Autodesk Fusion 360 part; units mm, degrees
(part 3 of 4)
sketch "Sketch5" plane through (0, 20, 0) normal (0, 1, 0) x (-1, 0, 0)
  line L0 (-11, 35) -> (-11, 37.5)
  line L1 (-11, 37.5) -> (-8.5, 37.5)
  line L2 (-8.5, 37.5) -> (-8.5, 35)
  line L3 (-8.5, 35) -> (-11, 35)
  line L4 (2.5, 35) -> (2.5, 37.5)
  line L5 (2.5, 37.5) -> (5, 37.5)
  line L6 (5, 37.5) -> (5, 35)
  line L7 (5, 35) -> (2.5, 35)
  line L8 (95, -45) -> (95, 155)
  line L9 (95, 155) -> (-95, 155)
  line L10 (-95, 155) -> (-95, -45)
  line L11 (-95, -45) -> (95, -45)
  line L12 (-63.1566, 125.0807) -> (-65.6424, 118.6138)
  line L13 (-65.6424, 118.6138) -> (-72.4858, 117.5331)
  line L14 (-72.4858, 117.5331) -> (-76.8434, 122.9193)
  line L15 (-76.8434, 122.9193) -> (-74.3576, 129.3862)
  line L16 (-74.3576, 129.3862) -> (-67.5142, 130.4669)
  line L17 (-67.5142, 130.4669) -> (-63.1566, 125.0807)
  line L18 (-63.1566, 93.0807) -> (-65.6424, 86.6138)
  line L19 (-65.6424, 86.6138) -> (-72.4858, 85.5331)
  line L20 (-72.4858, 85.5331) -> (-76.8434, 90.9193)
  line L21 (-76.8434, 90.9193) -> (-74.3576, 97.3862)
  line L22 (-74.3576, 97.3862) -> (-67.5142, 98.4669)
  line L23 (-67.5142, 98.4669) -> (-63.1566, 93.0807)
  line L24 (-63.1566, 61.0807) -> (-65.6424, 54.6138)
  line L25 (-65.6424, 54.6138) -> (-72.4858, 53.5331)
  line L26 (-72.4858, 53.5331) -> (-76.8434, 58.9193)
  line L27 (-76.8434, 58.9193) -> (-74.3576, 65.3862)
  line L28 (-74.3576, 65.3862) -> (-67.5142, 66.4669)
  line L29 (-67.5142, 66.4669) -> (-63.1566, 61.0807)
  line L30 (-63.1566, 29.0807) -> (-65.6424, 22.6138)
  line L31 (-65.6424, 22.6138) -> (-72.4858, 21.5331)
  line L32 (-72.4858, 21.5331) -> (-76.8434, 26.9193)
  line L33 (-76.8434, 26.9193) -> (-74.3576, 33.3862)
  line L34 (-74.3576, 33.3862) -> (-67.5142, 34.4669)
  line L35 (-67.5142, 34.4669) -> (-63.1566, 29.0807)
  line L36 (-63.1566, -2.9193) -> (-65.6424, -9.3862)
  line L37 (-65.6424, -9.3862) -> (-72.4858, -10.4669)
  line L38 (-72.4858, -10.4669) -> (-76.8434, -5.0807)
  line L39 (-76.8434, -5.0807) -> (-74.3576, 1.3862)
  line L40 (-74.3576, 1.3862) -> (-67.5142, 2.4669)
  line L41 (-67.5142, 2.4669) -> (-63.1566, -2.9193)
  line L42 (-49.8233, 141.0807) -> (-52.3091, 134.6138)
  line L43 (-52.3091, 134.6138) -> (-59.1525, 133.5331)
  line L44 (-59.1525, 133.5331) -> (-63.5101, 138.9193)
  line L45 (-63.5101, 138.9193) -> (-61.0243, 145.3862)
  line L46 (-61.0243, 145.3862) -> (-54.1809, 146.4669)
  line L47 (-54.1809, 146.4669) -> (-49.8233, 141.0807)
  line L48 (-49.8233, 109.0807) -> (-52.3091, 102.6138)
  line L49 (-52.3091, 102.6138) -> (-59.1525, 101.5331)
  line L50 (-59.1525, 101.5331) -> (-63.5101, 106.9193)
  line L51 (-63.5101, 106.9193) -> (-61.0243, 113.3862)
  line L52 (-61.0243, 113.3862) -> (-54.1809, 114.4669)
  line L53 (-54.1809, 114.4669) -> (-49.8233, 109.0807)
  line L54 (-49.8233, 77.0807) -> (-52.3091, 70.6138)
  line L55 (-52.3091, 70.6138) -> (-59.1525, 69.5331)
  line L56 (-59.1525, 69.5331) -> (-63.5101, 74.9193)
  line L57 (-63.5101, 74.9193) -> (-61.0243, 81.3862)
  line L58 (-61.0243, 81.3862) -> (-54.1809, 82.4669)
  line L59 (-54.1809, 82.4669) -> (-49.8233, 77.0807)
  line L60 (-49.8233, 45.0807) -> (-52.3091, 38.6138)
  line L61 (-52.3091, 38.6138) -> (-59.1525, 37.5331)
  line L62 (-59.1525, 37.5331) -> (-63.5101, 42.9193)
  line L63 (-63.5101, 42.9193) -> (-61.0243, 49.3862)
  line L64 (-61.0243, 49.3862) -> (-54.1809, 50.4669)
  line L65 (-54.1809, 50.4669) -> (-49.8233, 45.0807)
  line L66 (-49.8233, 13.0807) -> (-52.3091, 6.6138)
  line L67 (-52.3091, 6.6138) -> (-59.1525, 5.5331)
  line L68 (-59.1525, 5.5331) -> (-63.5101, 10.9193)
  line L69 (-63.5101, 10.9193) -> (-61.0243, 17.3862)
  line L70 (-61.0243, 17.3862) -> (-54.1809, 18.4669)
  line L71 (-54.1809, 18.4669) -> (-49.8233, 13.0807)
  line L72 (-49.8233, -18.9193) -> (-52.3091, -25.3862)
  line L73 (-52.3091, -25.3862) -> (-59.1525, -26.4669)
  line L74 (-59.1525, -26.4669) -> (-63.5101, -21.0807)
  line L75 (-63.5101, -21.0807) -> (-61.0243, -14.6138)
  line L76 (-61.0243, -14.6138) -> (-54.1809, -13.5331)
  line L77 (-54.1809, -13.5331) -> (-49.8233, -18.9193)
  line L78 (-36.4899, 125.0807) -> (-38.9757, 118.6138)
  line L79 (-38.9757, 118.6138) -> (-45.8191, 117.5331)
  line L80 (-45.8191, 117.5331) -> (-50.1767, 122.9193)
  line L81 (-50.1767, 122.9193) -> (-47.6909, 129.3862)
  line L82 (-47.6909, 129.3862) -> (-40.8475, 130.4669)
  line L83 (-40.8475, 130.4669) -> (-36.4899, 125.0807)
  line L84 (-36.4899, 93.0807) -> (-38.9757, 86.6138)
  line L85 (-38.9757, 86.6138) -> (-45.8191, 85.5331)
  line L86 (-45.8191, 85.5331) -> (-50.1767, 90.9193)
  line L87 (-50.1767, 90.9193) -> (-47.6909, 97.3862)
  line L88 (-47.6909, 97.3862) -> (-40.8475, 98.4669)
  line L89 (-40.8475, 98.4669) -> (-36.4899, 93.0807)
  line L90 (-36.4899, 61.0807) -> (-38.9757, 54.6138)
  line L91 (-38.9757, 54.6138) -> (-45.8191, 53.5331)
  line L92 (-45.8191, 53.5331) -> (-50.1767, 58.9193)
  line L93 (-50.1767, 58.9193) -> (-47.6909, 65.3862)
  line L94 (-47.6909, 65.3862) -> (-40.8475, 66.4669)
  line L95 (-40.8475, 66.4669) -> (-36.4899, 61.0807)
  line L96 (-36.4899, 29.0807) -> (-38.9757, 22.6138)
  line L97 (-38.9757, 22.6138) -> (-45.8191, 21.5331)
  line L98 (-45.8191, 21.5331) -> (-50.1767, 26.9193)
  line L99 (-50.1767, 26.9193) -> (-47.6909, 33.3862)
  line L100 (-47.6909, 33.3862) -> (-40.8475, 34.4669)
  line L101 (-40.8475, 34.4669) -> (-36.4899, 29.0807)
  line L102 (-36.4899, -2.9193) -> (-38.9757, -9.3862)
  line L103 (-38.9757, -9.3862) -> (-45.8191, -10.4669)
  line L104 (-45.8191, -10.4669) -> (-50.1767, -5.0807)
  line L105 (-50.1767, -5.0807) -> (-47.6909, 1.3862)
  line L106 (-47.6909, 1.3862) -> (-40.8475, 2.4669)
  line L107 (-40.8475, 2.4669) -> (-36.4899, -2.9193)
  line L108 (-23.1566, 141.0807) -> (-25.6424, 134.6138)
  line L109 (-25.6424, 134.6138) -> (-32.4858, 133.5331)
  line L110 (-32.4858, 133.5331) -> (-36.8434, 138.9193)
  line L111 (-36.8434, 138.9193) -> (-34.3576, 145.3862)
  line L112 (-34.3576, 145.3862) -> (-27.5142, 146.4669)
  line L113 (-27.5142, 146.4669) -> (-23.1566, 141.0807)
  line L114 (-23.1566, 109.0807) -> (-25.6424, 102.6138)
  line L115 (-25.6424, 102.6138) -> (-32.4858, 101.5331)
  line L116 (-32.4858, 101.5331) -> (-36.8434, 106.9193)
  line L117 (-36.8434, 106.9193) -> (-34.3576, 113.3862)
  line L118 (-34.3576, 113.3862) -> (-27.5142, 114.4669)
  line L119 (-27.5142, 114.4669) -> (-23.1566, 109.0807)
  line L120 (-23.1566, 77.0807) -> (-25.6424, 70.6138)
  line L121 (-25.6424, 70.6138) -> (-32.4858, 69.5331)
  line L122 (-32.4858, 69.5331) -> (-36.8434, 74.9193)
  line L123 (-36.8434, 74.9193) -> (-34.3576, 81.3862)
  line L124 (-34.3576, 81.3862) -> (-27.5142, 82.4669)
  line L125 (-27.5142, 82.4669) -> (-23.1566, 77.0807)
  line L126 (-23.1566, 45.0807) -> (-25.6424, 38.6138)
  line L127 (-25.6424, 38.6138) -> (-32.4858, 37.5331)
  line L128 (-32.4858, 37.5331) -> (-36.8434, 42.9193)
  line L129 (-36.8434, 42.9193) -> (-34.3576, 49.3862)
  line L130 (-34.3576, 49.3862) -> (-27.5142, 50.4669)
  line L131 (-27.5142, 50.4669) -> (-23.1566, 45.0807)
  line L132 (-23.1566, 13.0807) -> (-25.6424, 6.6138)
  line L133 (-25.6424, 6.6138) -> (-32.4858, 5.5331)
  line L134 (-32.4858, 5.5331) -> (-36.8434, 10.9193)
  line L135 (-36.8434, 10.9193) -> (-34.3576, 17.3862)
  line L136 (-34.3576, 17.3862) -> (-27.5142, 18.4669)
  line L137 (-27.5142, 18.4669) -> (-23.1566, 13.0807)
  line L138 (-23.1566, -18.9193) -> (-25.6424, -25.3862)
  line L139 (-25.6424, -25.3862) -> (-32.4858, -26.4669)
  line L140 (-32.4858, -26.4669) -> (-36.8434, -21.0807)
  line L141 (-36.8434, -21.0807) -> (-34.3576, -14.6138)
  line L142 (-34.3576, -14.6138) -> (-27.5142, -13.5331)
  line L143 (-27.5142, -13.5331) -> (-23.1566, -18.9193)
  line L144 (-9.8233, 125.0807) -> (-12.3091, 118.6138)
  line L145 (-12.3091, 118.6138) -> (-19.1525, 117.5331)
  line L146 (-19.1525, 117.5331) -> (-23.5101, 122.9193)
  line L147 (-23.5101, 122.9193) -> (-21.0243, 129.3862)
  line L148 (-21.0243, 129.3862) -> (-14.1809, 130.4669)
  line L149 (-14.1809, 130.4669) -> (-9.8233, 125.0807)
  line L150 (-9.8233, 93.0807) -> (-12.3091, 86.6138)
  line L151 (-12.3091, 86.6138) -> (-19.1525, 85.5331)
  line L152 (-19.1525, 85.5331) -> (-23.5101, 90.9193)
  line L153 (-23.5101, 90.9193) -> (-21.0243, 97.3862)
  line L154 (-21.0243, 97.3862) -> (-14.1809, 98.4669)
  line L155 (-14.1809, 98.4669) -> (-9.8233, 93.0807)
  line L156 (-9.8233, 61.0807) -> (-12.3091, 54.6138)
  line L157 (-12.3091, 54.6138) -> (-19.1525, 53.5331)
  line L158 (-19.1525, 53.5331) -> (-23.5101, 58.9193)
  line L159 (-23.5101, 58.9193) -> (-21.0243, 65.3862)
  line L160 (-21.0243, 65.3862) -> (-14.1809, 66.4669)
  line L161 (-14.1809, 66.4669) -> (-9.8233, 61.0807)
  line L162 (-9.8233, 29.0807) -> (-12.3091, 22.6138)
  line L163 (-12.3091, 22.6138) -> (-19.1525, 21.5331)
  line L164 (-19.1525, 21.5331) -> (-23.5101, 26.9193)
  line L165 (-23.5101, 26.9193) -> (-21.0243, 33.3862)
  line L166 (-21.0243, 33.3862) -> (-14.1809, 34.4669)
  line L167 (-14.1809, 34.4669) -> (-9.8233, 29.0807)
  line L168 (-9.8233, -2.9193) -> (-12.3091, -9.3862)
  line L169 (-12.3091, -9.3862) -> (-19.1525, -10.4669)
  line L170 (-19.1525, -10.4669) -> (-23.5101, -5.0807)
  line L171 (-23.5101, -5.0807) -> (-21.0243, 1.3862)
  line L172 (-21.0243, 1.3862) -> (-14.1809, 2.4669)
  line L173 (-14.1809, 2.4669) -> (-9.8233, -2.9193)
  line L174 (-0.8475, 146.4669) -> (3.5101, 141.0807)
  line L175 (3.5101, 141.0807) -> (1.0243, 134.6138)
  line L176 (1.0243, 134.6138) -> (-5.8191, 133.5331)
  line L177 (-5.8191, 133.5331) -> (-10.1767, 138.9193)
  line L178 (-10.1767, 138.9193) -> (-7.6909, 145.3862)
  line L179 (-7.6909, 145.3862) -> (-0.8475, 146.4669)
  line L180 (-0.8475, 114.4669) -> (3.5101, 109.0807)
  line L181 (3.5101, 109.0807) -> (1.0243, 102.6138)
  line L182 (1.0243, 102.6138) -> (-5.8191, 101.5331)
  line L183 (-5.8191, 101.5331) -> (-10.1767, 106.9193)
  line L184 (-10.1767, 106.9193) -> (-7.6909, 113.3862)
  line L185 (-7.6909, 113.3862) -> (-0.8475, 114.4669)
  line L186 (-0.8475, 82.4669) -> (3.5101, 77.0807)
  line L187 (3.5101, 77.0807) -> (1.0243, 70.6138)
  line L188 (1.0243, 70.6138) -> (-5.8191, 69.5331)
  line L189 (-5.8191, 69.5331) -> (-10.1767, 74.9193)
  line L190 (-10.1767, 74.9193) -> (-7.6909, 81.3862)
  line L191 (-7.6909, 81.3862) -> (-0.8475, 82.4669)
  line L192 (-0.8475, 50.4669) -> (3.5101, 45.0807)
  line L193 (3.5101, 45.0807) -> (1.0243, 38.6138)
  line L194 (1.0243, 38.6138) -> (-5.8191, 37.5331)
  line L195 (-5.8191, 37.5331) -> (-10.1767, 42.9193)
  line L196 (-10.1767, 42.9193) -> (-7.6909, 49.3862)
  line L197 (-7.6909, 49.3862) -> (-0.8475, 50.4669)
  line L198 (-0.8475, 18.4669) -> (3.5101, 13.0807)
  line L199 (3.5101, 13.0807) -> (1.0243, 6.6138)
  line L200 (1.0243, 6.6138) -> (-5.8191, 5.5331)
  line L201 (-5.8191, 5.5331) -> (-10.1767, 10.9193)
  line L202 (-10.1767, 10.9193) -> (-7.6909, 17.3862)
  line L203 (-7.6909, 17.3862) -> (-0.8475, 18.4669)
  line L204 (-0.8475, -13.5331) -> (3.5101, -18.9193)
  line L205 (3.5101, -18.9193) -> (1.0243, -25.3862)
  line L206 (1.0243, -25.3862) -> (-5.8191, -26.4669)
  line L207 (-5.8191, -26.4669) -> (-10.1767, -21.0807)
  line L208 (-10.1767, -21.0807) -> (-7.6909, -14.6138)
  line L209 (-7.6909, -14.6138) -> (-0.8475, -13.5331)
  line L210 (12.4858, 130.4669) -> (16.8434, 125.0807)
  line L211 (16.8434, 125.0807) -> (14.3576, 118.6138)
  line L212 (14.3576, 118.6138) -> (7.5142, 117.5331)
  line L213 (7.5142, 117.5331) -> (3.1566, 122.9193)
  line L214 (3.1566, 122.9193) -> (5.6424, 129.3862)
  line L215 (5.6424, 129.3862) -> (12.4858, 130.4669)
  line L216 (12.4858, 98.4669) -> (16.8434, 93.0807)
  line L217 (16.8434, 93.0807) -> (14.3576, 86.6138)
  line L218 (14.3576, 86.6138) -> (7.5142, 85.5331)
  line L219 (7.5142, 85.5331) -> (3.1566, 90.9193)
  line L220 (3.1566, 90.9193) -> (5.6424, 97.3862)
  line L221 (5.6424, 97.3862) -> (12.4858, 98.4669)
  line L222 (12.4858, 66.4669) -> (16.8434, 61.0807)
  line L223 (16.8434, 61.0807) -> (14.3576, 54.6138)
  line L224 (14.3576, 54.6138) -> (7.5142, 53.5331)
  line L225 (7.5142, 53.5331) -> (3.1566, 58.9193)
  line L226 (3.1566, 58.9193) -> (5.6424, 65.3862)
  line L227 (5.6424, 65.3862) -> (12.4858, 66.4669)
  line L228 (12.4858, 34.4669) -> (16.8434, 29.0807)
  line L229 (16.8434, 29.0807) -> (14.3576, 22.6138)
  line L230 (14.3576, 22.6138) -> (7.5142, 21.5331)
  line L231 (7.5142, 21.5331) -> (3.1566, 26.9193)
  line L232 (3.1566, 26.9193) -> (5.6424, 33.3862)
  line L233 (5.6424, 33.3862) -> (12.4858, 34.4669)
  line L234 (12.4858, 2.4669) -> (16.8434, -2.9193)
  line L235 (16.8434, -2.9193) -> (14.3576, -9.3862)
  line L236 (14.3576, -9.3862) -> (7.5142, -10.4669)
  line L237 (7.5142, -10.4669) -> (3.1566, -5.0807)
  line L238 (3.1566, -5.0807) -> (5.6424, 1.3862)
  line L239 (5.6424, 1.3862) -> (12.4858, 2.4669)
  line L240 (25.8191, 146.4669) -> (30.1767, 141.0807)
  line L241 (30.1767, 141.0807) -> (27.6909, 134.6138)
  line L242 (27.6909, 134.6138) -> (20.8475, 133.5331)
  line L243 (20.8475, 133.5331) -> (16.4899, 138.9193)
  line L244 (16.4899, 138.9193) -> (18.9757, 145.3862)
  line L245 (18.9757, 145.3862) -> (25.8191, 146.4669)
  line L246 (25.8191, 114.4669) -> (30.1767, 109.0807)
  line L247 (30.1767, 109.0807) -> (27.6909, 102.6138)
  line L248 (27.6909, 102.6138) -> (20.8475, 101.5331)
  line L249 (20.8475, 101.5331) -> (16.4899, 106.9193)
  line L250 (16.4899, 106.9193) -> (18.9757, 113.3862)
  line L251 (18.9757, 113.3862) -> (25.8191, 114.4669)
  line L252 (25.8191, 82.4669) -> (30.1767, 77.0807)
  line L253 (30.1767, 77.0807) -> (27.6909, 70.6138)
  line L254 (27.6909, 70.6138) -> (20.8475, 69.5331)
  line L255 (20.8475, 69.5331) -> (16.4899, 74.9193)
  line L256 (16.4899, 74.9193) -> (18.9757, 81.3862)
  line L257 (18.9757, 81.3862) -> (25.8191, 82.4669)
  line L258 (25.8191, 50.4669) -> (30.1767, 45.0807)
  line L259 (30.1767, 45.0807) -> (27.6909, 38.6138)
  line L260 (27.6909, 38.6138) -> (20.8475, 37.5331)
  line L261 (20.8475, 37.5331) -> (16.4899, 42.9193)
  line L262 (16.4899, 42.9193) -> (18.9757, 49.3862)
  line L263 (18.9757, 49.3862) -> (25.8191, 50.4669)
  line L264 (25.8191, 18.4669) -> (30.1767, 13.0807)
  line L265 (30.1767, 13.0807) -> (27.6909, 6.6138)
  line L266 (27.6909, 6.6138) -> (20.8475, 5.5331)
  line L267 (20.8475, 5.5331) -> (16.4899, 10.9193)
  line L268 (16.4899, 10.9193) -> (18.9757, 17.3862)
  line L269 (18.9757, 17.3862) -> (25.8191, 18.4669)
  line L270 (25.8191, -13.5331) -> (30.1767, -18.9193)
  line L271 (30.1767, -18.9193) -> (27.6909, -25.3862)
  line L272 (27.6909, -25.3862) -> (20.8475, -26.4669)
  line L273 (20.8475, -26.4669) -> (16.4899, -21.0807)
  line L274 (16.4899, -21.0807) -> (18.9757, -14.6138)
  line L275 (18.9757, -14.6138) -> (25.8191, -13.5331)
  line L276 (39.1525, 130.4669) -> (43.5101, 125.0807)
  line L277 (43.5101, 125.0807) -> (41.0243, 118.6138)
  line L278 (41.0243, 118.6138) -> (34.1809, 117.5331)
  line L279 (34.1809, 117.5331) -> (29.8233, 122.9193)
  line L280 (29.8233, 122.9193) -> (32.3091, 129.3862)
  line L281 (32.3091, 129.3862) -> (39.1525, 130.4669)
  line L282 (39.1525, 98.4669) -> (43.5101, 93.0807)
  line L283 (43.5101, 93.0807) -> (41.0243, 86.6138)
  line L284 (41.0243, 86.6138) -> (34.1809, 85.5331)
  line L285 (34.1809, 85.5331) -> (29.8233, 90.9193)
  line L286 (29.8233, 90.9193) -> (32.3091, 97.3862)
  line L287 (32.3091, 97.3862) -> (39.1525, 98.4669)
  line L288 (39.1525, 66.4669) -> (43.5101, 61.0807)
  line L289 (43.5101, 61.0807) -> (41.0243, 54.6138)
  line L290 (41.0243, 54.6138) -> (34.1809, 53.5331)
  line L291 (34.1809, 53.5331) -> (29.8233, 58.9193)
  line L292 (29.8233, 58.9193) -> (32.3091, 65.3862)
  line L293 (32.3091, 65.3862) -> (39.1525, 66.4669)
  line L294 (39.1525, 34.4669) -> (43.5101, 29.0807)
  line L295 (43.5101, 29.0807) -> (41.0243, 22.6138)
  line L296 (41.0243, 22.6138) -> (34.1809, 21.5331)
  line L297 (34.1809, 21.5331) -> (29.8233, 26.9193)
  line L298 (29.8233, 26.9193) -> (32.3091, 33.3862)
  line L299 (32.3091, 33.3862) -> (39.1525, 34.4669)
  line L300 (39.1525, 2.4669) -> (43.5101, -2.9193)
  line L301 (43.5101, -2.9193) -> (41.0243, -9.3862)
  line L302 (41.0243, -9.3862) -> (34.1809, -10.4669)
  line L303 (34.1809, -10.4669) -> (29.8233, -5.0807)
  line L304 (29.8233, -5.0807) -> (32.3091, 1.3862)
  line L305 (32.3091, 1.3862) -> (39.1525, 2.4669)
  line L306 (52.4858, 146.4669) -> (56.8434, 141.0807)
  line L307 (56.8434, 141.0807) -> (54.3576, 134.6138)
  line L308 (54.3576, 134.6138) -> (47.5142, 133.5331)
  line L309 (47.5142, 133.5331) -> (43.1566, 138.9193)
  line L310 (43.1566, 138.9193) -> (45.6424, 145.3862)
  line L311 (45.6424, 145.3862) -> (52.4858, 146.4669)
  line L312 (52.4858, 114.4669) -> (56.8434, 109.0807)
  line L313 (56.8434, 109.0807) -> (54.3576, 102.6138)
  line L314 (54.3576, 102.6138) -> (47.5142, 101.5331)
  line L315 (47.5142, 101.5331) -> (43.1566, 106.9193)
  line L316 (43.1566, 106.9193) -> (45.6424, 113.3862)
  line L317 (45.6424, 113.3862) -> (52.4858, 114.4669)
  line L318 (52.4858, 82.4669) -> (56.8434, 77.0807)
  line L319 (56.8434, 77.0807) -> (54.3576, 70.6138)
  line L320 (54.3576, 70.6138) -> (47.5142, 69.5331)
  line L321 (47.5142, 69.5331) -> (43.1566, 74.9193)
  line L322 (43.1566, 74.9193) -> (45.6424, 81.3862)
  line L323 (45.6424, 81.3862) -> (52.4858, 82.4669)
  line L324 (52.4858, 50.4669) -> (56.8434, 45.0807)
  line L325 (56.8434, 45.0807) -> (54.3576, 38.6138)
  line L326 (54.3576, 38.6138) -> (47.5142, 37.5331)
  line L327 (47.5142, 37.5331) -> (43.1566, 42.9193)
  line L328 (43.1566, 42.9193) -> (45.6424, 49.3862)
  line L329 (45.6424, 49.3862) -> (52.4858, 50.4669)
  line L330 (52.4858, 18.4669) -> (56.8434, 13.0807)
  line L331 (56.8434, 13.0807) -> (54.3576, 6.6138)
  line L332 (54.3576, 6.6138) -> (47.5142, 5.5331)
  line L333 (47.5142, 5.5331) -> (43.1566, 10.9193)
  line L334 (43.1566, 10.9193) -> (45.6424, 17.3862)
  line L335 (45.6424, 17.3862) -> (52.4858, 18.4669)
  line L336 (47.5142, -26.4669) -> (43.1566, -21.0807)
  line L337 (43.1566, -21.0807) -> (45.6424, -14.6138)
  line L338 (45.6424, -14.6138) -> (52.4858, -13.5331)
  line L339 (52.4858, -13.5331) -> (56.8434, -18.9193)
  line L340 (56.8434, -18.9193) -> (54.3576, -25.3862)
  line L341 (54.3576, -25.3862) -> (47.5142, -26.4669)
  line L342 (52.4858, 2.4669) -> (56.8434, -2.9193)
  line L343 (56.8434, -2.9193) -> (54.3576, -9.3862)
  line L344 (54.3576, -9.3862) -> (47.5142, -10.4669)
  line L345 (47.5142, -10.4669) -> (43.1566, -5.0807)
  line L346 (43.1566, -5.0807) -> (45.6424, 1.3862)
  line L347 (45.6424, 1.3862) -> (52.4858, 2.4669)
  line L348 (52.4858, 34.4669) -> (56.8434, 29.0807)
  line L349 (56.8434, 29.0807) -> (54.3576, 22.6138)
  line L350 (54.3576, 22.6138) -> (47.5142, 21.5331)
  line L351 (47.5142, 21.5331) -> (43.1566, 26.9193)
  line L352 (43.1566, 26.9193) -> (45.6424, 33.3862)
  line L353 (45.6424, 33.3862) -> (52.4858, 34.4669)
  line L354 (52.4858, 66.4669) -> (56.8434, 61.0807)
  line L355 (56.8434, 61.0807) -> (54.3576, 54.6138)
  line L356 (54.3576, 54.6138) -> (47.5142, 53.5331)
  line L357 (47.5142, 53.5331) -> (43.1566, 58.9193)
  line L358 (43.1566, 58.9193) -> (45.6424, 65.3862)
  line L359 (45.6424, 65.3862) -> (52.4858, 66.4669)
  line L360 (52.4858, 98.4669) -> (56.8434, 93.0807)
  line L361 (56.8434, 93.0807) -> (54.3576, 86.6138)
  line L362 (54.3576, 86.6138) -> (47.5142, 85.5331)
  line L363 (47.5142, 85.5331) -> (43.1566, 90.9193)
  line L364 (43.1566, 90.9193) -> (45.6424, 97.3862)
  line L365 (45.6424, 97.3862) -> (52.4858, 98.4669)
  line L366 (52.4858, 130.4669) -> (56.8434, 125.0807)
  line L367 (56.8434, 125.0807) -> (54.3576, 118.6138)
  line L368 (54.3576, 118.6138) -> (47.5142, 117.5331)
  line L369 (47.5142, 117.5331) -> (43.1566, 122.9193)
  line L370 (43.1566, 122.9193) -> (45.6424, 129.3862)
  line L371 (45.6424, 129.3862) -> (52.4858, 130.4669)
  line L372 (39.1525, -13.5331) -> (43.5101, -18.9193)
  line L373 (43.5101, -18.9193) -> (41.0243, -25.3862)
  line L374 (41.0243, -25.3862) -> (34.1809, -26.4669)
  line L375 (34.1809, -26.4669) -> (29.8233, -21.0807)
  line L376 (29.8233, -21.0807) -> (32.3091, -14.6138)
  line L377 (32.3091, -14.6138) -> (39.1525, -13.5331)
  line L378 (39.1525, 18.4669) -> (43.5101, 13.0807)
  line L379 (43.5101, 13.0807) -> (41.0243, 6.6138)
  line L380 (41.0243, 6.6138) -> (34.1809, 5.5331)
  line L381 (34.1809, 5.5331) -> (29.8233, 10.9193)
  line L382 (29.8233, 10.9193) -> (32.3091, 17.3862)
  line L383 (32.3091, 17.3862) -> (39.1525, 18.4669)
  line L384 (39.1525, 50.4669) -> (43.5101, 45.0807)
  line L385 (43.5101, 45.0807) -> (41.0243, 38.6138)
  line L386 (41.0243, 38.6138) -> (34.1809, 37.5331)
  line L387 (34.1809, 37.5331) -> (29.8233, 42.9193)
  line L388 (29.8233, 42.9193) -> (32.3091, 49.3862)
  line L389 (32.3091, 49.3862) -> (39.1525, 50.4669)
  line L390 (39.1525, 82.4669) -> (43.5101, 77.0807)
  line L391 (43.5101, 77.0807) -> (41.0243, 70.6138)
  line L392 (41.0243, 70.6138) -> (34.1809, 69.5331)
  line L393 (34.1809, 69.5331) -> (29.8233, 74.9193)
  line L394 (29.8233, 74.9193) -> (32.3091, 81.3862)
  line L395 (32.3091, 81.3862) -> (39.1525, 82.4669)
  line L396 (39.1525, 114.4669) -> (43.5101, 109.0807)
  line L397 (43.5101, 109.0807) -> (41.0243, 102.6138)
  line L398 (41.0243, 102.6138) -> (34.1809, 101.5331)
  line L399 (34.1809, 101.5331) -> (29.8233, 106.9193)
  line L400 (29.8233, 106.9193) -> (32.3091, 113.3862)
  line L401 (32.3091, 113.3862) -> (39.1525, 114.4669)
  line L402 (39.1525, 146.4669) -> (43.5101, 141.0807)
  line L403 (43.5101, 141.0807) -> (41.0243, 134.6138)
  line L404 (41.0243, 134.6138) -> (34.1809, 133.5331)
  line L405 (34.1809, 133.5331) -> (29.8233, 138.9193)
  line L406 (29.8233, 138.9193) -> (32.3091, 145.3862)
  line L407 (32.3091, 145.3862) -> (39.1525, 146.4669)
  line L408 (25.8191, 2.4669) -> (30.1767, -2.9193)
  line L409 (30.1767, -2.9193) -> (27.6909, -9.3862)
  line L410 (27.6909, -9.3862) -> (20.8475, -10.4669)
  line L411 (20.8475, -10.4669) -> (16.4899, -5.0807)
  line L412 (16.4899, -5.0807) -> (18.9757, 1.3862)
  line L413 (18.9757, 1.3862) -> (25.8191, 2.4669)
  line L414 (25.8191, 34.4669) -> (30.1767, 29.0807)
  line L415 (30.1767, 29.0807) -> (27.6909, 22.6138)
  line L416 (27.6909, 22.6138) -> (20.8475, 21.5331)
  line L417 (20.8475, 21.5331) -> (16.4899, 26.9193)
  line L418 (16.4899, 26.9193) -> (18.9757, 33.3862)
  line L419 (18.9757, 33.3862) -> (25.8191, 34.4669)
  line L420 (25.8191, 66.4669) -> (30.1767, 61.0807)
  line L421 (30.1767, 61.0807) -> (27.6909, 54.6138)
  line L422 (27.6909, 54.6138) -> (20.8475, 53.5331)
  line L423 (20.8475, 53.5331) -> (16.4899, 58.9193)
  line L424 (16.4899, 58.9193) -> (18.9757, 65.3862)
  line L425 (18.9757, 65.3862) -> (25.8191, 66.4669)
  line L426 (25.8191, 98.4669) -> (30.1767, 93.0807)
  line L427 (30.1767, 93.0807) -> (27.6909, 86.6138)
  line L428 (27.6909, 86.6138) -> (20.8475, 85.5331)
  line L429 (20.8475, 85.5331) -> (16.4899, 90.9193)
  line L430 (16.4899, 90.9193) -> (18.9757, 97.3862)
  line L431 (18.9757, 97.3862) -> (25.8191, 98.4669)
  line L432 (25.8191, 130.4669) -> (30.1767, 125.0807)
  line L433 (30.1767, 125.0807) -> (27.6909, 118.6138)
  line L434 (27.6909, 118.6138) -> (20.8475, 117.5331)
  line L435 (20.8475, 117.5331) -> (16.4899, 122.9193)
  line L436 (16.4899, 122.9193) -> (18.9757, 129.3862)
  line L437 (18.9757, 129.3862) -> (25.8191, 130.4669)
  line L438 (12.4858, -13.5331) -> (16.8434, -18.9193)
  line L439 (16.8434, -18.9193) -> (14.3576, -25.3862)
  line L440 (14.3576, -25.3862) -> (7.5142, -26.4669)
  line L441 (7.5142, -26.4669) -> (3.1566, -21.0807)
  line L442 (3.1566, -21.0807) -> (5.6424, -14.6138)
  line L443 (5.6424, -14.6138) -> (12.4858, -13.5331)
  line L444 (12.4858, 18.4669) -> (16.8434, 13.0807)
  line L445 (16.8434, 13.0807) -> (14.3576, 6.6138)
  line L446 (14.3576, 6.6138) -> (7.5142, 5.5331)
  line L447 (7.5142, 5.5331) -> (3.1566, 10.9193)
  line L448 (3.1566, 10.9193) -> (5.6424, 17.3862)
  line L449 (5.6424, 17.3862) -> (12.4858, 18.4669)
  line L450 (12.4858, 50.4669) -> (16.8434, 45.0807)
  line L451 (16.8434, 45.0807) -> (14.3576, 38.6138)
  line L452 (14.3576, 38.6138) -> (7.5142, 37.5331)
  line L453 (7.5142, 37.5331) -> (3.1566, 42.9193)
  line L454 (3.1566, 42.9193) -> (5.6424, 49.3862)
  line L455 (5.6424, 49.3862) -> (12.4858, 50.4669)
  line L456 (12.4858, 82.4669) -> (16.8434, 77.0807)
  line L457 (16.8434, 77.0807) -> (14.3576, 70.6138)
  line L458 (14.3576, 70.6138) -> (7.5142, 69.5331)
  line L459 (7.5142, 69.5331) -> (3.1566, 74.9193)
  line L460 (3.1566, 74.9193) -> (5.6424, 81.3862)
  line L461 (5.6424, 81.3862) -> (12.4858, 82.4669)
  line L462 (12.4858, 114.4669) -> (16.8434, 109.0807)
  line L463 (16.8434, 109.0807) -> (14.3576, 102.6138)
  line L464 (14.3576, 102.6138) -> (7.5142, 101.5331)
  line L465 (7.5142, 101.5331) -> (3.1566, 106.9193)
  line L466 (3.1566, 106.9193) -> (5.6424, 113.3862)
  line L467 (5.6424, 113.3862) -> (12.4858, 114.4669)
  line L468 (12.4858, 146.4669) -> (16.8434, 141.0807)
  line L469 (16.8434, 141.0807) -> (14.3576, 134.6138)
  line L470 (14.3576, 134.6138) -> (7.5142, 133.5331)
  line L471 (7.5142, 133.5331) -> (3.1566, 138.9193)
  line L472 (3.1566, 138.9193) -> (5.6424, 145.3862)
  line L473 (5.6424, 145.3862) -> (12.4858, 146.4669)
  line L474 (-0.8475, 2.4669) -> (3.5101, -2.9193)
  line L475 (3.5101, -2.9193) -> (1.0243, -9.3862)
  line L476 (1.0243, -9.3862) -> (-5.8191, -10.4669)
  line L477 (-5.8191, -10.4669) -> (-10.1767, -5.0807)
  line L478 (-10.1767, -5.0807) -> (-7.6909, 1.3862)
  line L479 (-7.6909, 1.3862) -> (-0.8475, 2.4669)
  line L480 (-0.8475, 34.4669) -> (3.5101, 29.0807)
  line L481 (3.5101, 29.0807) -> (1.0243, 22.6138)
  line L482 (1.0243, 22.6138) -> (-5.8191, 21.5331)
  line L483 (-5.8191, 21.5331) -> (-10.1767, 26.9193)
  line L484 (-10.1767, 26.9193) -> (-7.6909, 33.3862)
  line L485 (-7.6909, 33.3862) -> (-0.8475, 34.4669)
  line L486 (-0.8475, 66.4669) -> (3.5101, 61.0807)
  line L487 (3.5101, 61.0807) -> (1.0243, 54.6138)
  line L488 (1.0243, 54.6138) -> (-5.8191, 53.5331)
  line L489 (-5.8191, 53.5331) -> (-10.1767, 58.9193)
  line L490 (-10.1767, 58.9193) -> (-7.6909, 65.3862)
  line L491 (-7.6909, 65.3862) -> (-0.8475, 66.4669)
  line L492 (-0.8475, 98.4669) -> (3.5101, 93.0807)
  line L493 (3.5101, 93.0807) -> (1.0243, 86.6138)
  line L494 (1.0243, 86.6138) -> (-5.8191, 85.5331)
  line L495 (-5.8191, 85.5331) -> (-10.1767, 90.9193)
  line L496 (-10.1767, 90.9193) -> (-7.6909, 97.3862)
  line L497 (-7.6909, 97.3862) -> (-0.8475, 98.4669)
  line L498 (-0.8475, 130.4669) -> (3.5101, 125.0807)
  line L499 (3.5101, 125.0807) -> (1.0243, 118.6138)
  line L500 (1.0243, 118.6138) -> (-5.8191, 117.5331)
  line L501 (-5.8191, 117.5331) -> (-10.1767, 122.9193)
  line L502 (-10.1767, 122.9193) -> (-7.6909, 129.3862)
  line L503 (-7.6909, 129.3862) -> (-0.8475, 130.4669)
  line L504 (-14.1809, -13.5331) -> (-9.8233, -18.9193)
  line L505 (-9.8233, -18.9193) -> (-12.3091, -25.3862)
  line L506 (-12.3091, -25.3862) -> (-19.1525, -26.4669)
  line L507 (-19.1525, -26.4669) -> (-23.5101, -21.0807)
  line L508 (-23.5101, -21.0807) -> (-21.0243, -14.6138)
  line L509 (-21.0243, -14.6138) -> (-14.1809, -13.5331)
  line L510 (-9.8233, 13.0807) -> (-12.3091, 6.6138)
  line L511 (-12.3091, 6.6138) -> (-19.1525, 5.5331)
  line L512 (-19.1525, 5.5331) -> (-23.5101, 10.9193)
  line L513 (-23.5101, 10.9193) -> (-21.0243, 17.3862)
  line L514 (-21.0243, 17.3862) -> (-14.1809, 18.4669)
  line L515 (-14.1809, 18.4669) -> (-9.8233, 13.0807)
  line L516 (-9.8233, 45.0807) -> (-12.3091, 38.6138)
  line L517 (-12.3091, 38.6138) -> (-19.1525, 37.5331)
  line L518 (-19.1525, 37.5331) -> (-23.5101, 42.9193)
  line L519 (-23.5101, 42.9193) -> (-21.0243, 49.3862)
  line L520 (-21.0243, 49.3862) -> (-14.1809, 50.4669)
  line L521 (-14.1809, 50.4669) -> (-9.8233, 45.0807)
  line L522 (-9.8233, 77.0807) -> (-12.3091, 70.6138)
  line L523 (-12.3091, 70.6138) -> (-19.1525, 69.5331)
  line L524 (-19.1525, 69.5331) -> (-23.5101, 74.9193)
  line L525 (-23.5101, 74.9193) -> (-21.0243, 81.3862)
  line L526 (-21.0243, 81.3862) -> (-14.1809, 82.4669)
  line L527 (-14.1809, 82.4669) -> (-9.8233, 77.0807)
  line L528 (-9.8233, 109.0807) -> (-12.3091, 102.6138)
  line L529 (-12.3091, 102.6138) -> (-19.1525, 101.5331)
  line L530 (-19.1525, 101.5331) -> (-23.5101, 106.9193)
  line L531 (-23.5101, 106.9193) -> (-21.0243, 113.3862)
  line L532 (-21.0243, 113.3862) -> (-14.1809, 114.4669)
  line L533 (-14.1809, 114.4669) -> (-9.8233, 109.0807)
  line L534 (-9.8233, 141.0807) -> (-12.3091, 134.6138)
  line L535 (-12.3091, 134.6138) -> (-19.1525, 133.5331)
  line L536 (-19.1525, 133.5331) -> (-23.5101, 138.9193)
  line L537 (-23.5101, 138.9193) -> (-21.0243, 145.3862)
  line L538 (-21.0243, 145.3862) -> (-14.1809, 146.4669)
  line L539 (-14.1809, 146.4669) -> (-9.8233, 141.0807)
  line L540 (-23.1566, -2.9193) -> (-25.6424, -9.3862)
  line L541 (-25.6424, -9.3862) -> (-32.4858, -10.4669)
  line L542 (-32.4858, -10.4669) -> (-36.8434, -5.0807)
  line L543 (-36.8434, -5.0807) -> (-34.3576, 1.3862)
  line L544 (-34.3576, 1.3862) -> (-27.5142, 2.4669)
  line L545 (-27.5142, 2.4669) -> (-23.1566, -2.9193)
  line L546 (-23.1566, 29.0807) -> (-25.6424, 22.6138)
  line L547 (-25.6424, 22.6138) -> (-32.4858, 21.5331)
  line L548 (-32.4858, 21.5331) -> (-36.8434, 26.9193)
  line L549 (-36.8434, 26.9193) -> (-34.3576, 33.3862)
  line L550 (-34.3576, 33.3862) -> (-27.5142, 34.4669)
  line L551 (-27.5142, 34.4669) -> (-23.1566, 29.0807)
  line L552 (-23.1566, 61.0807) -> (-25.6424, 54.6138)
  line L553 (-25.6424, 54.6138) -> (-32.4858, 53.5331)
  line L554 (-32.4858, 53.5331) -> (-36.8434, 58.9193)
  line L555 (-36.8434, 58.9193) -> (-34.3576, 65.3862)
  line L556 (-34.3576, 65.3862) -> (-27.5142, 66.4669)
  line L557 (-27.5142, 66.4669) -> (-23.1566, 61.0807)
  line L558 (-23.1566, 93.0807) -> (-25.6424, 86.6138)
  line L559 (-25.6424, 86.6138) -> (-32.4858, 85.5331)
  line L560 (-32.4858, 85.5331) -> (-36.8434, 90.9193)
  line L561 (-36.8434, 90.9193) -> (-34.3576, 97.3862)
  line L562 (-34.3576, 97.3862) -> (-27.5142, 98.4669)
  line L563 (-27.5142, 98.4669) -> (-23.1566, 93.0807)
  line L564 (-23.1566, 125.0807) -> (-25.6424, 118.6138)
  line L565 (-25.6424, 118.6138) -> (-32.4858, 117.5331)
  line L566 (-32.4858, 117.5331) -> (-36.8434, 122.9193)
  line L567 (-36.8434, 122.9193) -> (-34.3576, 129.3862)
  line L568 (-34.3576, 129.3862) -> (-27.5142, 130.4669)
  line L569 (-27.5142, 130.4669) -> (-23.1566, 125.0807)
  line L570 (-36.4899, -18.9193) -> (-38.9757, -25.3862)
  line L571 (-38.9757, -25.3862) -> (-45.8191, -26.4669)
  line L572 (-45.8191, -26.4669) -> (-50.1767, -21.0807)
  line L573 (-50.1767, -21.0807) -> (-47.6909, -14.6138)
  line L574 (-47.6909, -14.6138) -> (-40.8475, -13.5331)
  line L575 (-40.8475, -13.5331) -> (-36.4899, -18.9193)
  line L576 (-36.4899, 13.0807) -> (-38.9757, 6.6138)
  line L577 (-38.9757, 6.6138) -> (-45.8191, 5.5331)
  line L578 (-45.8191, 5.5331) -> (-50.1767, 10.9193)
  line L579 (-50.1767, 10.9193) -> (-47.6909, 17.3862)
  line L580 (-47.6909, 17.3862) -> (-40.8475, 18.4669)
  line L581 (-40.8475, 18.4669) -> (-36.4899, 13.0807)
  line L582 (-36.4899, 45.0807) -> (-38.9757, 38.6138)
  line L583 (-38.9757, 38.6138) -> (-45.8191, 37.5331)
  line L584 (-45.8191, 37.5331) -> (-50.1767, 42.9193)
  line L585 (-50.1767, 42.9193) -> (-47.6909, 49.3862)
  line L586 (-47.6909, 49.3862) -> (-40.8475, 50.4669)
  line L587 (-40.8475, 50.4669) -> (-36.4899, 45.0807)
  line L588 (-36.4899, 77.0807) -> (-38.9757, 70.6138)
  line L589 (-38.9757, 70.6138) -> (-45.8191, 69.5331)
  line L590 (-45.8191, 69.5331) -> (-50.1767, 74.9193)
  line L591 (-50.1767, 74.9193) -> (-47.6909, 81.3862)
  line L592 (-47.6909, 81.3862) -> (-40.8475, 82.4669)
  line L593 (-40.8475, 82.4669) -> (-36.4899, 77.0807)
  line L594 (-36.4899, 109.0807) -> (-38.9757, 102.6138)
  line L595 (-38.9757, 102.6138) -> (-45.8191, 101.5331)
  line L596 (-45.8191, 101.5331) -> (-50.1767, 106.9193)
  line L597 (-50.1767, 106.9193) -> (-47.6909, 113.3862)
  line L598 (-47.6909, 113.3862) -> (-40.8475, 114.4669)
  line L599 (-40.8475, 114.4669) -> (-36.4899, 109.0807)
  line L600 (-36.4899, 141.0807) -> (-38.9757, 134.6138)
  line L601 (-38.9757, 134.6138) -> (-45.8191, 133.5331)
  line L602 (-45.8191, 133.5331) -> (-50.1767, 138.9193)
  line L603 (-50.1767, 138.9193) -> (-47.6909, 145.3862)
  line L604 (-47.6909, 145.3862) -> (-40.8475, 146.4669)
  line L605 (-40.8475, 146.4669) -> (-36.4899, 141.0807)
  line L606 (-49.8233, -2.9193) -> (-52.3091, -9.3862)
  line L607 (-52.3091, -9.3862) -> (-59.1525, -10.4669)
  line L608 (-59.1525, -10.4669) -> (-63.5101, -5.0807)
  line L609 (-63.5101, -5.0807) -> (-61.0243, 1.3862)
  line L610 (-61.0243, 1.3862) -> (-54.1809, 2.4669)
  line L611 (-54.1809, 2.4669) -> (-49.8233, -2.9193)
  line L612 (-49.8233, 29.0807) -> (-52.3091, 22.6138)
  line L613 (-52.3091, 22.6138) -> (-59.1525, 21.5331)
  line L614 (-59.1525, 21.5331) -> (-63.5101, 26.9193)
  line L615 (-63.5101, 26.9193) -> (-61.0243, 33.3862)
  line L616 (-61.0243, 33.3862) -> (-54.1809, 34.4669)
  line L617 (-54.1809, 34.4669) -> (-49.8233, 29.0807)
  line L618 (-49.8233, 61.0807) -> (-52.3091, 54.6138)
  line L619 (-52.3091, 54.6138) -> (-59.1525, 53.5331)
  line L620 (-59.1525, 53.5331) -> (-63.5101, 58.9193)
  line L621 (-63.5101, 58.9193) -> (-61.0243, 65.3862)
  line L622 (-61.0243, 65.3862) -> (-54.1809, 66.4669)
  line L623 (-54.1809, 66.4669) -> (-49.8233, 61.0807)
  line L624 (-49.8233, 93.0807) -> (-52.3091, 86.6138)
  line L625 (-52.3091, 86.6138) -> (-59.1525, 85.5331)
  line L626 (-59.1525, 85.5331) -> (-63.5101, 90.9193)
  line L627 (-63.5101, 90.9193) -> (-61.0243, 97.3862)
  line L628 (-61.0243, 97.3862) -> (-54.1809, 98.4669)
  line L629 (-54.1809, 98.4669) -> (-49.8233, 93.0807)
  line L630 (-49.8233, 125.0807) -> (-52.3091, 118.6138)
  line L631 (-52.3091, 118.6138) -> (-59.1525, 117.5331)
  line L632 (-59.1525, 117.5331) -> (-63.5101, 122.9193)
  line L633 (-63.5101, 122.9193) -> (-61.0243, 129.3862)
  line L634 (-61.0243, 129.3862) -> (-54.1809, 130.4669)
  line L635 (-54.1809, 130.4669) -> (-49.8233, 125.0807)
  line L636 (-63.1566, -18.9193) -> (-65.6424, -25.3862)
  line L637 (-65.6424, -25.3862) -> (-72.4858, -26.4669)
  line L638 (-72.4858, -26.4669) -> (-76.8434, -21.0807)
  line L639 (-76.8434, -21.0807) -> (-74.3576, -14.6138)
  line L640 (-74.3576, -14.6138) -> (-67.5142, -13.5331)
  line L641 (-67.5142, -13.5331) -> (-63.1566, -18.9193)
  line L642 (-63.1566, 13.0807) -> (-65.6424, 6.6138)
  line L643 (-65.6424, 6.6138) -> (-72.4858, 5.5331)
  line L644 (-72.4858, 5.5331) -> (-76.8434, 10.9193)
  line L645 (-76.8434, 10.9193) -> (-74.3576, 17.3862)
  line L646 (-74.3576, 17.3862) -> (-67.5142, 18.4669)
  line L647 (-67.5142, 18.4669) -> (-63.1566, 13.0807)
  line L648 (-63.1566, 45.0807) -> (-65.6424, 38.6138)
  line L649 (-65.6424, 38.6138) -> (-72.4858, 37.5331)
  line L650 (-72.4858, 37.5331) -> (-76.8434, 42.9193)
  line L651 (-76.8434, 42.9193) -> (-74.3576, 49.3862)
  line L652 (-74.3576, 49.3862) -> (-67.5142, 50.4669)
  line L653 (-67.5142, 50.4669) -> (-63.1566, 45.0807)
  line L654 (-63.1566, 77.0807) -> (-65.6424, 70.6138)
  line L655 (-65.6424, 70.6138) -> (-72.4858, 69.5331)
  line L656 (-72.4858, 69.5331) -> (-76.8434, 74.9193)
  line L657 (-76.8434, 74.9193) -> (-74.3576, 81.3862)
  line L658 (-74.3576, 81.3862) -> (-67.5142, 82.4669)
  line L659 (-67.5142, 82.4669) -> (-63.1566, 77.0807)
  line L660 (-63.1566, 109.0807) -> (-65.6424, 102.6138)
  line L661 (-65.6424, 102.6138) -> (-72.4858, 101.5331)
  line L662 (-72.4858, 101.5331) -> (-76.8434, 106.9193)
  line L663 (-76.8434, 106.9193) -> (-74.3576, 113.3862)
  line L664 (-74.3576, 113.3862) -> (-67.5142, 114.4669)
  line L665 (-67.5142, 114.4669) -> (-63.1566, 109.0807)
  line L666 (-63.1566, 141.0807) -> (-65.6424, 134.6138)
  line L667 (-65.6424, 134.6138) -> (-72.4858, 133.5331)
  line L668 (-72.4858, 133.5331) -> (-76.8434, 138.9193)
  line L669 (-76.8434, 138.9193) -> (-74.3576, 145.3862)
  line L670 (-74.3576, 145.3862) -> (-67.5142, 146.4669)
  line L671 (-67.5142, 146.4669) -> (-63.1566, 141.0807)
  line L672 (2, 85) -> (4.5, 85)
  line L673 (4.5, 85) -> (4.5, 82.5)
  line L674 (4.5, 82.5) -> (2, 82.5)
  line L675 (2, 82.5) -> (2, 85)
  line L676 (-11.0662, 85.0201) -> (-8.5662, 85.0201)
  line L677 (-8.5662, 85.0201) -> (-8.5662, 82.5201)
  line L678 (-8.5662, 82.5201) -> (-11.0662, 82.5201)
  line L679 (-11.0662, 82.5201) -> (-11.0662, 85.0201)
  dimension "d29" = 2.5
  dimension "d30" = 2.5
  dimension "d31" = 2.5
  dimension "d32" = 2.5
  constraint horizontal L672
  constraint vertical L673
  constraint horizontal L674
  constraint vertical L675
  constraint horizontal L676
  constraint vertical L677
  constraint horizontal L678
  constraint vertical L679
  measures "d29" distance of L672.start L672.end
  measures "d30" distance of L672.start L674.end
  measures "d31" distance of L676.start L676.end
  measures "d32" distance of L676.start L678.end
extrude "Extrude6" add sketch "Sketch5" along normal blind 70 contours L672 L673 L674 L675 | L676 L677 L678 L679 bodies 1
sketch "Sketch6" plane through (0, 90, 0) normal (0, 1, 0) x (-1, 0, 0)
  line L0 (-11, 35) -> (-8.5, 35)
  line L1 (-8.5, 35) -> (-8.5, 37.5)
  line L2 (-8.5, 37.5) -> (-11, 37.5)
  line L3 (-11, 37.5) -> (-11, 35)
  line L4 (-30, 35) -> (25, 35)
  line L5 (25, 35) -> (25, 85)
  line L6 (25, 85) -> (-30, 85)
  line L7 (-30, 85) -> (-30, 35)
  dimension "d35" = 50
  constraint horizontal L4
  constraint vertical L5
  constraint horizontal L6
  constraint vertical L7
  measures "d35" distance of L4.start L6.end
sketch "Sketch7" plane through (0, 90, 0) normal (0, 1, 0) x (-1, 0, 0)
  line L0 (-11, 35) -> (-8.5027, 35)
  line L1 (-8.5027, 35) -> (-8.5027, 38.142)
  line L2 (-8.5027, 38.142) -> (-11, 38.142)
  line L3 (-11, 38.142) -> (-11, 35)
  constraint horizontal L0
  constraint vertical L1
  constraint horizontal L2
  constraint vertical L3
extrude "Extrude7" add sketch "Sketch6" sketch "Sketch7" along normal blind 10 separate body contours L1 L2 L3 L4 L5 L6 L7 of sketch 2 makes body 2
sketch "Sketch8" plane through (0, 0, -49) normal (0, 0, -1) x (-1, 0, 0)
  line L0 (-99, 250) -> (-99, 18)
  line L1 (-99, 18) -> (99, 18)
  line L2 (99, 18) -> (99, 250)
  line L3 (99, 250) -> (-99, 250)
  line L4 (-90, 240, 2.1) -> (90, 240, 2.1)
  line L5 (90, 240, 2.1) -> (90, 237.8787, -0.0213)
  line L6 (90, 237.8787, -0.0213) -> (-90, 237.8787, -0.0213)
  line L7 (-90, 237.8787, -0.0213) -> (-90, 240, 2.1)
  dimension "d38" = 3
extrude "Extrude8" cut sketch "Sketch8" along normal blind 10 contours L4 L5 L6 L7 in plane through (0, 118.9504, 69.95) normal (0, 0.707108, 0.707106) bodies 1
pattern_linear "R-Pattern2" count 15 spacing 14.2857 along (0, -1, 0) count 3 spacing 2.5 along (1, 0, 0) of "Extrude8"
sketch "Sketch9" plane through (0, 0, 159) normal (0, 0, 1) x (1, 0, 0)
  line L0 (99, 250) -> (-95, 250)
  line L1 (-95, 250) -> (-95, 20)
  line L2 (-95, 20) -> (-99, 20)
  line L3 (-99, 20) -> (-99, 18)
  line L4 (-99, 18) -> (99, 18)
  line L5 (99, 18) -> (99, 250)
  line L6 (-90, 240, 3.1) -> (90, 240, 3.1)
  line L7 (90, 240, 3.1) -> (90, 237.8787, 0.9787)
  line L8 (90, 237.8787, 0.9787) -> (-90, 237.8787, 0.9787)
  line L9 (-90, 237.8787, 0.9787) -> (-90, 240, 3.1)
  dimension "d45" = 180
  dimension "d46" = 3
extrude "Extrude9" cut sketch "Sketch9" along normal blind 10 contours L6 L7 L8 L9 in plane through (0, 118.45, 40.55) normal (0, 0.707107, -0.707107) bodies 1
pattern_linear "R-Pattern3" count 15 spacing 14.2857 along (0, -1, 0) of "Extrude9"
sketch "Sketch10" plane through (99, 0, 0) normal (1, 0, 0) x (0, 0, -1)
  line L0 (-159, 250) -> (-159, 18)
  line L1 (-159, 18) -> (49, 18)
  line L2 (49, 18) -> (49, 250)
  line L3 (49, 250) -> (-159, 250)
  line L4 (-150, 239.1213, 2.1213) -> (40, 239.1213, 2.1213)
  line L5 (40, 239.1213, 2.1213) -> (40, 237, 0)
  line L6 (40, 237) -> (-150, 237)
  line L7 (-150, 237, 0) -> (-150, 239.1213, 2.1213)
  dimension "d53" = 190
  dimension "d54" = 3
extrude "Extrude10" cut sketch "Sketch10" along normal blind 10 contours L4 L5 L6 L7 in plane through (-19.5, 118.5, 0) normal (-0.707107, 0.707107, 0) bodies 1
pattern_linear "R-Pattern4" count 15 spacing 14.2857 along (0, -1, 0) of "Extrude10"
delete_face "DeleteFace1" 5 faces at (-100, 96.6667, 156.6667) (-98.3333, 96.6667, 160) (-98, 20, 159.6667) (-95, 96.6667, 159.6667) (-99.3333, 96.6667, 155) on bodies 1
sketch "Sketch11" plane through (-99, 0, 0) normal (-1, 0, 0) x (0, 0, 1)
  line L0 (159, 18) -> (159, 250)
  line L1 (159, 250) -> (-49, 250)
  line L2 (-49, 250) -> (-49, 18)
  line L3 (-49, 18) -> (159, 18)
  line L4 (-10, 209.1213, 2.1213) -> (120, 209.1213, 2.1213)
  line L5 (120, 209.1213, 2.1213) -> (120, 207, 0)
  line L6 (120, 207) -> (-10, 207)
  line L7 (-10, 207, 0) -> (-10, 209.1213, 2.1213)
  dimension "d61" = 3
extrude "Extrude11" cut sketch "Sketch11" along normal blind 10 contours L4 L5 L6 L7 in plane through (4.5, 103.5, 0) normal (0.707107, 0.707107, 0) bodies 1
pattern_linear "R-Pattern5" count 10 spacing 16.6667 along (0, -1, 0) of "Extrude11"
sketch "Sketch12" plane through (0, 100, 0) normal (0, 1, 0) x (-1, 0, 0)
  line L0 (-8.5027, 37.5) -> (-8.5, 37.5)
  line L1 (-8.5, 37.5) -> (-8.5, 35)
  line L2 (-8.5, 35) -> (25, 35)
  line L3 (25, 35) -> (25, 85)
  line L4 (25, 85) -> (-30, 85)
  line L5 (-30, 85) -> (-30, 35)
  line L6 (-30, 35) -> (-8.5027, 35)
  line L7 (-8.5027, 35) -> (-8.5027, 37.5)
  line L8 (-30, 85) -> (-60, 85)
  line L9 (-60, 85) -> (-60, 35)
  line L10 (-60, 35) -> (-30, 35)
  line L11 (-30, 35) -> (-30, 85)
  line L12 (25, 35) -> (55, 35)
  line L13 (55, 35) -> (55, 85)
  line L14 (55, 85) -> (25, 85)
  line L15 (25, 85) -> (25, 35)
  line L16 (-60, 35) -> (55, 35)
  line L17 (55, 35) -> (55, 5)
  line L18 (55, 5) -> (-60, 5)
  line L19 (-60, 5) -> (-60, 35)
  line L20 (-60, 85) -> (55, 85)
  line L21 (55, 85) -> (55, 115)
  line L22 (55, 115) -> (-60, 115)
  line L23 (-60, 115) -> (-60, 85)
  dimension "d68" = 30
  dimension "d69" = 50
  dimension "d70" = 30
  dimension "d71" = 50
  dimension "d72" = 115
  dimension "d73" = 30
  dimension "d74" = 115
  dimension "d75" = 30
  constraint horizontal L8
  constraint vertical L9
  constraint horizontal L10
  constraint vertical L11
  constraint coincident L4.end L5.start
  constraint horizontal L12
  constraint vertical L13
  constraint horizontal L14
  constraint vertical L15
  constraint coincident L2.end L3.start
  constraint horizontal L16
  constraint vertical L17
  constraint horizontal L18
  constraint vertical L19
  constraint horizontal L20
  constraint vertical L21
  constraint horizontal L22
  constraint vertical L23
  measures "d68" distance of L4.end L8.end
  measures "d69" distance of L4.end L5.end
  measures "d70" distance of L2.end L12.end
  measures "d71" distance of L2.end L3.end
  measures "d72" distance of L9.end L12.end
  measures "d73" distance of L9.end L18.end
  measures "d74" distance of L8.end L13.end
  measures "d75" distance of L8.end L22.end
extrude "Extrude12" add sketch "Sketch12" against normal blind 10 contours L2 L6 L10 L12 L16 L17 L18 L19 | L5 L8 L9 L10 L11 L16 L20 | L3 L12 L13 L14 L15 L16 L20 | L4 L8 L14 L20 L21 L22 L23 bodies 1 2
sketch "Sketch13" plane through (-99, 0, 0) normal (-1, 0, 0) x (0, 0, 1)
  line L0 (-10, 57) -> (-10, 61.2426)
  line L1 (-10, 61.2426) -> (120, 61.2426)
  line L2 (120, 61.2426) -> (120, 57)
  line L3 (120, 57) -> (-10, 57)
  line L4 (-10, 73.6667) -> (-10, 77.9093)
  line L5 (-10, 77.9093) -> (120, 77.9093)
  line L6 (120, 77.9093) -> (120, 73.6667)
  line L7 (120, 73.6667) -> (-10, 73.6667)
  line L8 (-10, 90.3333) -> (-10, 94.576)
  line L9 (-10, 94.576) -> (120, 94.576)
  line L10 (120, 94.576) -> (120, 90.3333)
  line L11 (120, 90.3333) -> (-10, 90.3333)
  line L12 (-10, 107) -> (-10, 111.2426)
  line L13 (-10, 111.2426) -> (120, 111.2426)
  line L14 (120, 111.2426) -> (120, 107)
  line L15 (120, 107) -> (-10, 107)
  line L16 (-10, 123.6667) -> (-10, 127.9093)
  line L17 (-10, 127.9093) -> (120, 127.9093)
  line L18 (120, 127.9093) -> (120, 123.6667)
  line L19 (120, 123.6667) -> (-10, 123.6667)
  line L20 (-10, 140.3333) -> (-10, 144.576)
  line L21 (-10, 144.576) -> (120, 144.576)
  line L22 (120, 144.576) -> (120, 140.3333)
  line L23 (120, 140.3333) -> (-10, 140.3333)
  line L24 (-10, 157) -> (-10, 161.2426)
  line L25 (-10, 161.2426) -> (120, 161.2426)
  line L26 (120, 161.2426) -> (120, 157)
  line L27 (120, 157) -> (-10, 157)
  line L28 (-10, 173.6667) -> (-10, 177.9093)
  line L29 (-10, 177.9093) -> (120, 177.9093)
  line L30 (120, 177.9093) -> (120, 173.6667)
  line L31 (120, 173.6667) -> (-10, 173.6667)
  line L32 (-10, 190.3333) -> (-10, 194.576)
  line L33 (-10, 194.576) -> (120, 194.576)
  line L34 (120, 194.576) -> (120, 190.3333)
  line L35 (120, 190.3333) -> (-10, 190.3333)
  line L36 (120, 211.2426) -> (120, 207)
  line L37 (120, 207) -> (-10, 207)
  line L38 (-10, 207) -> (-10, 211.2426)
  line L39 (-10, 211.2426) -> (120, 211.2426)
  line L40 (159, 18) -> (159, 250)
  line L41 (159, 250) -> (-49, 250)
  line L42 (-49, 250) -> (-49, 18)
  line L43 (-49, 18) -> (159, 18)
  line L44 (-30, 230, 20) -> (140, 230, 20)
  line L45 (140, 230, 20) -> (140, 40, 20)
  line L46 (140, 40, 20) -> (-30, 40, 20)
  line L47 (-30, 40, 20) -> (-30, 230, 20)
extrude "Extrude13" cut sketch "Sketch13" against normal blind 40 contours L44 L45 L46 L47 in plane through (-119, 0, 0) normal (-1, 0, 0) bodies 1
sketch "Sketch14" plane through (-99, 0, 0) normal (-1, 0, 0) x (0, 0, 1)
  line L0 (140, 230) -> (140, 40)
  line L1 (140, 40) -> (-30, 40)
  line L2 (-30, 40) -> (-30, 230)
  line L3 (-30, 230) -> (140, 230)
  line L4 (159, 18) -> (159, 250)
  line L5 (159, 250) -> (-49, 250)
  line L6 (-49, 250) -> (-49, 18)
  line L7 (-49, 18) -> (159, 18)
  line L8 (-30, 230) -> (140, 230)
  line L9 (140, 230) -> (140, 40)
  line L10 (140, 40) -> (-30, 40)
  line L11 (-30, 40) -> (-30, 230)
  constraint horizontal L8
  constraint vertical L9
  constraint horizontal L10
  constraint vertical L11
  constraint coincident L0.end L1.start
  constraint coincident L2.end L3.start
extrude "Extrude1'" add sketch "Sketch14" along normal blind 5 separate body contours L0 L1 L2 L3 L8 L9 L10 L11 makes body 3 in component "Component"
move_body "Move1" bodies 3 to x (1, 0, 0) y (0, 1, 0) z (0, 0, 1) at (20, 0, 0) in component "Component"
sketch "Sketch15" plane through (-164, 0, 0) normal (-1, 0, 0) x (0, 0, 1)
  line L0 (-30, 40) -> (140, 40)
  line L1 (140, 40) -> (140, 230)
  line L2 (140, 230) -> (-30, 230)
  line L3 (-30, 230) -> (-30, 40)
  line L4 (-5, 205.8787, -0.1213) -> (115, 205.8787, -0.1213)
  line L5 (115, 205.8787, -0.1213) -> (115, 208, 2)
  line L6 (115, 208, 2) -> (-5, 208, 2)
  line L7 (-5, 208, 2) -> (-5, 205.8787, -0.1213)
  dimension "d82" = 120
  dimension "d83" = 3
extrude "Extrude2'" cut sketch "Sketch15" against normal blind 10 contours L4 L5 L6 L7 in plane through (-61, 103, 0) normal (-0.707107, -0.707107, 0) sketch seen with x (1, 0, 0) y (0, 1, 0) z (0, 0, 1) at (80, 0, 0) bodies 3 in component "Component"
pattern_linear "R-Pattern1'" count 10 spacing 16.6667 along (0, -1, 0) of "Extrude2'" in component "Component"
sketch "Sketch16" plane through (0, 250, 0) normal (0, 1, 0) x (-1, 0, 0)
  line L0 (99, -49) -> (99, 159)
  line L1 (99, 159) -> (-99, 159)
  line L2 (-99, 159) -> (-99, -49)
  line L3 (-99, -49) -> (99, -49)
  line L4 (95, -45) -> (-95, -45)
  line L5 (-95, -45) -> (-95, 155)
  line L6 (-95, 155) -> (95, 155)
  line L7 (95, 155) -> (95, -45)
  line L8 (-99, -49) -> (99, -49)
  line L9 (99, -49) -> (99, 159)
  line L10 (99, 159) -> (-99, 159)
  line L11 (-99, 159) -> (-99, -49)
  constraint horizontal L8
  constraint vertical L9
  constraint horizontal L10
  constraint vertical L11
  constraint coincident L0.end L1.start
  constraint coincident L2.end L3.start
extrude "Extrude14" add sketch "Sketch16" along normal blind 5 separate body contours L4 L5 L6 L7 makes body 4
move_body "Move1'" bodies 4 to x (1, 0, 0) y (0, 1, 0) z (0, 0, 1) at (0, -5, 0)
sketch "Sketch17" plane through (0, 250, 0) normal (0, 1, 0) x (-1, 0, 0)
  line L0 (95, 155) -> (-95, 155)
  line L1 (-95, 155) -> (-95, -45)
  line L2 (-95, -45) -> (95, -45)
  line L3 (95, -45) -> (95, 155)
sketch "Sketch18" plane through (0, 250, 0) normal (0, 1, 0) x (-1, 0, 0)
  line L0 (99, -49) -> (90, -49)
  line L1 (90, -49) -> (90, -40)
  line L2 (90, -40) -> (99, -40)
  line L3 (99, -40) -> (99, -49)
  line L4 (-99, -49) -> (-90, -49)
  line L5 (-90, -49) -> (-90, -40)
  line L6 (-90, -40) -> (-99, -40)
  line L7 (-99, -40) -> (-99, -49)
  dimension "d92" = 9
  dimension "d93" = 9
  dimension "d94" = 9
  dimension "d95" = 9
  constraint horizontal L0
  constraint vertical L1
  constraint horizontal L2
  constraint vertical L3
  constraint horizontal L4
  constraint vertical L5
  constraint horizontal L6
  constraint vertical L7
  measures "d92" distance of L0.start L0.end
  measures "d93" distance of L0.start L2.end
  measures "d94" distance of L4.start L4.end
  measures "d95" distance of L4.start L6.end
extrude "Extrude15" add sketch "Sketch18" along normal blind 30 bodies 1 4